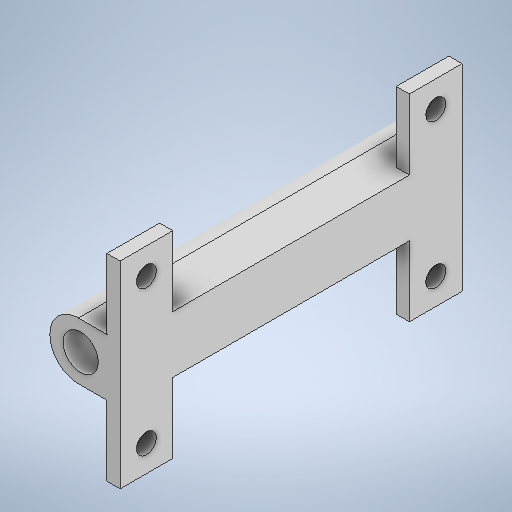
# Autodesk Inventor part: Axle Hold
Saved by Autodesk Inventor 2025 (Build 290162000, 162)
## iProperties
Created: 2024-11-04
Part Number: Axle Hold
Material: Generic
Document SubType Name: Modeling
Designer: liaco
Density: 1 g/cm^3
Appearance: Default
Author: liaco
Autodesk Inventor part; units mm, degrees
ref_plane "YZ Plane" through (0, 0, 0) normal (1, 0, 0) x (0, 1, 0)
ref_plane "XZ Plane" through (0, 0, 0) normal (0, 1, 0) x (-1, 0, 0)
ref_plane "XY Plane" through (0, 0, 0) normal (0, 0, 1) x (1, 0, 0)
sketch "Sketch1" plane through (0, 0, 0) normal (1, 0, 0) x (0, 1, 0)
  line L0 (-22.5, 39) -> (22.5, 39)
  line L1 (22.5, -39) -> (-22.5, -39)
  line L2 (-22.5, 39) -> (22.5, -39) construction
  line L3 (22.5, 39) -> (-22.5, -39) construction
  line L4 (22.5, 39) -> (22.5, -39)
  line L5 (-22.5, -39) -> (-22.5, 39)
  line L6 (22.5, 0) -> (-22.5, 0)
  point P0 (0, 0)
  point P1 (16.5, 33)
  point P2 (-16.5, 33)
  point P3 (16.5, -33)
  point P4 (-16.5, -33)
  dimension "d43" = 78
  dimension "d44" = 45
  dimension "d45" = 6
  dimension "d46" = 6
  dimension "d47" = 6
  dimension "d48" = 6
  constraints: 14 end point, 4 midpoint, 2 parallel, 2 symmetric about line, 1 horizontal, 1 perpendicular
  measures "d43" distance of L0.end L1.start
  measures "d44" distance of L0.start L0.end
  measures "d45" distance from line of L0 point (16.5, 33)
  measures "d46" distance from line of L0 point (-16.5, 33)
  measures "d47" distance from line of L5 point (-16.5, 33)
  measures "d48" distance from line of L4 point (16.5, 33)
extrude "Extrusion3" add sketch "Sketch1" along normal blind 3
hole "Hole3" at (0, 16.5, 33) at (0, 16.5, -33) at (0, -16.5, -33) at (0, -16.5, 33) direction (1, 0, 0) diameter 4.5 end through all clearance for "Flat Head Machine Screw" size "M4" standard "Ansi Metric M Profile"
sketch "Sketch4" plane through (0, 0, 0) normal (-1, 0, 0) x (0, 0, 1)
  line L0 (39, 22.5) -> (39, -22.5) projected
  line L1 (-39, -6.5) -> (39, -6.5)
  line L2 (39, -6.5) -> (39, 6.5)
  line L3 (39, 6.5) -> (-39, 6.5)
  line L4 (-39, 6.5) -> (-39, -6.5)
  line L5 (-39, -6.5) -> (39, 6.5) construction
  line L6 (39, -6.5) -> (-39, 6.5) construction
  point P0 (0, 0)
  dimension "d49" = 13
  constraints: 12 end point, 2 midpoint, 2 parallel, 1 horizontal, 1 perpendicular, 1 point on line
  measures "d49" distance between parallel lines of L3 L1
extrude "Extrusion4" add sketch "Sketch4" along normal blind 13
full round fillet "Full Round Fillet2" first side at (-4.3333, -6.5, -13) centre faces at (-13, 2.1667, -13) second side at (-4.3333, 6.5, 13)
sketch "Sketch5" plane through (0, -22.5, 39) normal (0, 0, 1) x (1, 0, 0)
  line L0 (0, 29) -> (-6.5, 29) projected
  point P0 (0, 22.5)
  point P1 (-6, 22.5)
  dimension "d52" = 6
  dimension "d53" = 6.5
  measures "d52" distance of point (0, 22.5) point (-6, 22.5)
  measures "d53" distance from line of L0 point (-6, 22.5)
hole "Hole4" at (-6, 0, 39) direction (0, 0, -1) diameter 8 end through all
sketch "Sketch6" plane through (3, 0, 0) normal (1, 0, 0) x (0, 0, -1)
  line L0 (39, 22.5) -> (-39, 22.5) projected
  line L1 (39, 6.5) -> (-39, 6.5) projected
  line L2 (-27, 22.5) -> (27, 22.5)
  line L3 (27, 22.5) -> (27, 6.5)
  line L4 (27, 6.5) -> (-27, 6.5)
  line L5 (-27, 6.5) -> (-27, 22.5)
  line L6 (-39, -22.5) -> (39, -22.5) projected
  line L7 (-27, -22.5) -> (27, -22.5)
  line L8 (27, -22.5) -> (27, -6.5)
  line L9 (27, -6.5) -> (-27, -6.5)
  line L10 (-27, -6.5) -> (-27, -22.5)
  line L11 (-39, -6.5) -> (39, -6.5) projected
  circle A0 centre (33, 16.5) radius 2.25 projected
  circle A1 centre (-33, 16.5) radius 2.25 projected
  point P0 (0, 0)
  point P1 (27, -22.5)
  dimension "d61" = 0
  dimension "d62" = 6
  dimension "d63" = 6
  constraints: 16 end point, 5 point on line, 4 parallel, 2 horizontal, 2 perpendicular
  measures "d61" distance between parallel lines of L11 L9
  measures "d62" distance from line of A0.centre L3
  measures "d63" distance from line of A1.centre L5
extrude "Extrusion5" cut sketch "Sketch6" against normal blind 10 contours L3 L1 L5 L0 | L10 L9 L8 L6
body "Solid2"
